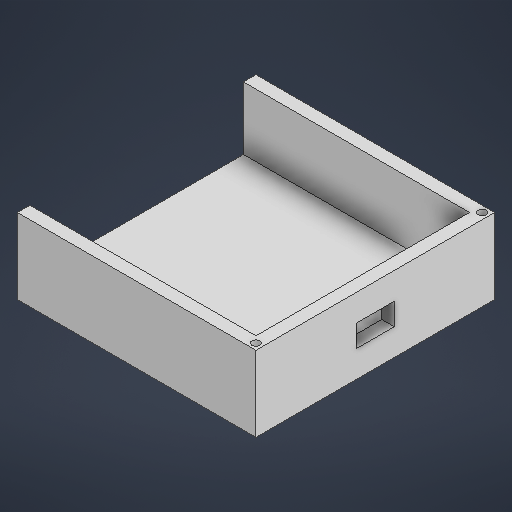
# Autodesk Inventor part: Caja_Bateria
Saved by Autodesk Inventor 2026 (Build 300175000, 175)
## iProperties
Created: 2025-11-03
Part Number: Caja_Bateria
Material: Generic
Document SubType Name: Modeling
Designer: Nicolás De Bruijn
Density: 1 g/cm^3
Appearance: Default
Author: Nicolás De Bruijn
Autodesk Inventor part; units mm, degrees
ref_plane "YZ Plane" through (0, 0, 0) normal (1, 0, 0) x (0, 1, 0)
ref_plane "XZ Plane" through (0, 0, 0) normal (0, 1, 0) x (-1, 0, 0)
ref_plane "XY Plane" through (0, 0, 0) normal (0, 0, 1) x (1, 0, 0)
sketch "Sketch4" plane through (0, 0, 0) normal (0, 1, 0) x (-1, 0, 0)
  line L0 (-47.5, -47.5) -> (47.5, -47.5)
  line L1 (47.5, -47.5) -> (47.5, 47.5)
  line L2 (47.5, 47.5) -> (-47.5, 47.5)
  line L3 (-47.5, 47.5) -> (-47.5, -47.5)
  line L4 (-47.5, -47.5) -> (47.5, 47.5) construction
  line L5 (47.5, -47.5) -> (-47.5, 47.5) construction
  point P0 (0, 0)
  dimension "d24" = 95
  dimension "d25" = 95
  constraints: 12 end point, 2 midpoint, 2 parallel, 1 horizontal, 1 perpendicular
  measures "d24" distance of L2.end L1.end
  measures "d25" distance of L1.end L0.end
extrude "Extrusion4" add sketch "Sketch4" along normal blind 5
sketch "Sketch5" plane through (0, 5, 0) normal (0, 1, 0) x (1, 0, 0)
  line L0 (-47.5, 47.5) -> (-47.5, -47.5) projected
  line L1 (-47.5, -42.5) -> (42.5, -42.5)
  line L2 (47.5, -47.5) -> (47.5, 47.5) projected
  line L3 (-47.5, -47.5) -> (47.5, -47.5) projected
  line L4 (42.5, -42.5) -> (42.5, 42.5)
  line L5 (-47.5, 42.5) -> (42.5, 42.5)
  line L6 (47.5, 47.5) -> (-47.5, 47.5) projected
  point P0 (0, 0)
  dimension "d28" = 5
  dimension "d29" = 5
  dimension "d30" = 5
  constraints: 6 end point, 2 point on line, 1 horizontal, 1 perpendicular, 1 vertical, 1 other
  measures "d28" distance between parallel lines of L1 L3
  measures "d29" distance between parallel lines of L2 L4
extrude "Extrusion5" add sketch "Sketch5" along normal blind 25 contours L6 L2 L3 L0 L1 L4 L5
sketch "Sketch6" plane through (0, 30, 0) normal (0, 1, 0) x (1, 0, 0)
  circle A0 centre (45, -45) radius 1.6
  circle A1 centre (45, 45) radius 1.6
  line L0 (47.5, -47.5) -> (47.5, 47.5) projected
  line L1 (-47.5, -47.5) -> (47.5, -47.5) projected
  line L2 (47.5, 47.5) -> (-47.5, 47.5) projected
  point P0 (0, 0)
  dimension "d33" = 3.2
  dimension "d34" = 3.2
  dimension "d35" = 2.5
  dimension "d36" = 2.5
  dimension "d37" = 2.5
  dimension "d38" = 2.5
  constraints: 2 centre point
  measures "d33" diameter of A0
  measures "d34" diameter of A1
  measures "d35" distance from line of L0 A0.centre
  measures "d36" distance from line of L1 A0.centre
  measures "d37" distance from line of L0 A1.centre
  measures "d38" distance from line of L2 A1.centre
extrude "Extrusion6" cut sketch "Sketch6" against normal blind 25
sketch "Sketch7" plane through (47.5, 0, 47.5) normal (1, 0, 0) x (0, 0, -1)
  line L0 (39.95, 19.4) -> (55.05, 19.4)
  line L1 (55.05, 19.4) -> (55.05, 10.6)
  line L2 (55.05, 10.6) -> (39.95, 10.6)
  line L3 (39.95, 10.6) -> (39.95, 19.4)
  line L4 (39.95, 19.4) -> (55.05, 10.6) construction
  line L5 (55.05, 19.4) -> (39.95, 10.6) construction
  line L6 (0, 0) -> (95, 0) projected
  line L7 (0, 30) -> (95, 30) projected
  line L8 (0, 0) -> (0, 30) projected
  line L9 (95, 0) -> (95, 30) projected
  point P0 (47.5, 0)
  point P1 (47.5, 15)
  dimension "d41" = 15.1
  dimension "d42" = 8.8
  dimension "d43" = 10.6
  dimension "d44" = 10.6
  dimension "d45" = 39.95
  dimension "d46" = 39.95
  constraints: 12 end point, 2 midpoint, 2 parallel, 1 horizontal, 1 perpendicular
  measures "d41" distance of L1.end L2.end
  measures "d42" distance of L0.end L1.end
  measures "d43" distance between parallel lines of L6 L2
  measures "d44" distance between parallel lines of L7 L0
  measures "d45" distance between parallel lines of L8 L3
  measures "d46" distance between parallel lines of L9 L1
extrude "Extrusion7" cut sketch "Sketch7" against normal blind 25 contours L0 L1 L2 L3
body "Solid2"
